Autodesk Fusion 360 part; units mm, degrees
note: some values were not read from the file. Chosen so that the rebuilt part matches the saved one: which face or edge a step refers to; which pieces of a blend or face edit are solid. Set by a fixed rule: which sketch regions a step uses.
(part 3 of 5)
sketch "スケッチ6" plane through (0, 0, 1.5) normal (0, 0, 1) x (-1, 0, 0)
  arc A0 (-32.0144, 97.3721) -> (-38.6662, 94.9272) centre (0, 0) ccw
  arc A1 (-26.3162, 95.431) -> (-32.0144, 97.3721) centre (-30.4528, 92.6222) ccw
  arc A2 (-26.3162, 95.431) -> (-25.9652, 94.9247) centre (0, 113.3) ccw
  arc A3 (-26.1835, 92.3551) -> (-25.9652, 94.9247) centre (-27.5978, 93.7693) ccw
  line L0 (-26.1835, 92.3551) -> (-32.3993, 86.1394)
  arc A4 (-35.2277, 86.1394) -> (-32.3993, 86.1394) centre (-33.8135, 87.5536) ccw
  line L1 (-35.2277, 86.1394) -> (-39.5548, 90.4665)
  arc A5 (-40.036, 92.519) -> (-39.5548, 90.4665) centre (-38.1406, 91.8807) ccw
  arc A6 (-40.036, 92.519) -> (-39.9088, 93.1825) centre (-42.4052, 93.3169) ccw
  arc A7 (-38.6662, 94.9272) -> (-39.9088, 93.1825) centre (-37.9117, 93.075) ccw
  line L2 (39.5548, 90.4665) -> (35.2277, 86.1394)
  arc A8 (32.3993, 86.1394) -> (35.2277, 86.1394) centre (33.8135, 87.5536) ccw
  line L3 (32.3993, 86.1394) -> (26.1835, 92.3551)
  arc A9 (25.9652, 94.9247) -> (26.1835, 92.3551) centre (27.5978, 93.7693) ccw
  arc A10 (25.9652, 94.9247) -> (26.3162, 95.431) centre (0, 113.3) ccw
  arc A11 (32.0144, 97.3721) -> (26.3162, 95.431) centre (30.4528, 92.6222) ccw
  arc A12 (38.6662, 94.9272) -> (32.0144, 97.3721) centre (0, 0) ccw
  arc A13 (39.9088, 93.1825) -> (38.6662, 94.9272) centre (37.9117, 93.075) ccw
  arc A14 (39.9088, 93.1825) -> (40.036, 92.519) centre (42.4052, 93.3169) ccw
  arc A15 (39.5548, 90.4665) -> (40.036, 92.519) centre (38.1406, 91.8807) ccw
  circle A16 centre (69.3456, -45.6575) radius 1.75
  circle A17 centre (-45.6575, -69.3456) radius 1.75
  circle A18 centre (-69.3456, 45.6575) radius 1.75
  circle A19 centre (69.3307, 45.6801) radius 1.75
  circle A20 centre (-93.3169, 42.4052) radius 1.75
  circle A21 centre (42.4052, -93.3169) radius 1.75
  circle A22 centre (93.3169, -42.4052) radius 1.75
  circle A23 centre (45.6801, -69.3307) radius 1.75
  circle A24 centre (-69.3307, -45.6801) radius 1.75
  circle A25 centre (-45.6801, 69.3307) radius 1.75
  circle A26 centre (45.6575, 69.3456) radius 1.75
  circle A27 centre (-93.3169, -42.4052) radius 1.75
  circle A28 centre (-42.4052, -93.3169) radius 1.75
  circle A29 centre (93.3169, 42.4052) radius 1.75
  circle A30 centre (39.2089, -15.5208) radius 1.75
  circle A31 centre (15.5208, -39.2089) radius 1.75
  circle A32 centre (26.1275, -49.8155) radius 1.75
  circle A33 centre (49.8155, -26.1275) radius 1.75
  circle A34 centre (-42.4052, 93.3169) radius 1.75
  circle A35 centre (-26.1275, 49.8155) radius 1.75
  arc A36 (-24.0851, 35.8083) -> (-23.3401, 43.4926) centre (-26.8756, 39.9571) ccw
  arc A37 (-24.0851, 35.8083) -> (-35.8083, 24.0851) centre (0, 0) ccw
  arc A38 (-43.4926, 23.3401) -> (-35.8083, 24.0851) centre (-39.9571, 26.8756) ccw
  line L4 (-43.4926, 23.3401) -> (-62.6322, 42.4797)
  arc A39 (-62.2927, 49.1749) -> (-62.6322, 42.4797) centre (-58.7571, 45.6394) ccw
  line L5 (-62.2927, 49.1749) -> (-49.1931, 62.2745)
  arc A40 (-42.122, 62.2745) -> (-49.1931, 62.2745) centre (-45.6575, 58.739) ccw
  line L6 (-42.122, 62.2745) -> (-23.3401, 43.4926)
  circle A41 centre (-49.8155, -26.1275) radius 1.75
  circle A42 centre (-49.8155, 26.1275) radius 1.75
  circle A43 centre (-15.5208, 39.2089) radius 1.75
  circle A44 centre (-26.1275, -49.8155) radius 1.75
  circle A45 centre (-39.2089, 15.5208) radius 1.75
  circle A46 centre (-15.5208, -39.2089) radius 1.75
  circle A47 centre (-39.2089, -15.5208) radius 1.75
  circle A48 centre (42.4052, 93.3169) radius 1.75
  arc A49 (17.125, 34.0956) -> (-17.125, 34.0956) centre (0, 0) ccw
  line L7 (17.125, 34.0956) -> (17.1965, 34.167)
  line L8 (17.1965, 34.167) -> (17.4152, 33.9483)
  arc A50 (33.9483, 17.4152) -> (17.4152, 33.9483) centre (0, 0) ccw
  line L9 (33.9483, 17.4152) -> (34.167, 17.1965)
  line L10 (34.167, 17.1965) -> (34.0956, 17.125)
  arc A51 (-34.0956, 17.125) -> (34.0956, 17.125) centre (0, 0) ccw
  line L11 (-34.0956, 17.125) -> (-34.167, 17.1965)
  line L12 (-34.167, 17.1965) -> (-33.9483, 17.4152)
  arc A52 (-17.4152, 33.9483) -> (-33.9483, 17.4152) centre (0, 0) ccw
  line L13 (-17.4152, 33.9483) -> (-17.1965, 34.167)
  line L14 (-17.1965, 34.167) -> (-17.125, 34.0956)
  line L15 (38.5865, 65.8101) -> (15.8059, 43.0296)
  arc A53 (10.9963, 41.7301) -> (15.8059, 43.0296) centre (12.2704, 46.5651) ccw
  arc A54 (10.9963, 41.7301) -> (-10.9963, 41.7301) centre (0, 0) ccw
  arc A55 (-15.8059, 43.0296) -> (-10.9963, 41.7301) centre (-12.2704, 46.5651) ccw
  line L16 (-15.8059, 43.0296) -> (-38.5865, 65.8101)
  arc A56 (-38.5865, 72.8811) -> (-38.5865, 65.8101) centre (-35.0509, 69.3456) ccw
  line L17 (-38.5865, 72.8811) -> (-24.7285, 86.7391)
  arc A57 (-18.3143, 87.2917) -> (-24.7285, 86.7391) centre (-21.193, 83.2035) ccw
  arc A58 (-18.3143, 87.2917) -> (18.3143, 87.2917) centre (0, 113.3) ccw
  arc A59 (24.7285, 86.7391) -> (18.3143, 87.2917) centre (21.193, 83.2035) ccw
  line L18 (24.7285, 86.7391) -> (38.5865, 72.8811)
  arc A60 (38.5865, 65.8101) -> (38.5865, 72.8811) centre (35.0509, 69.3456) ccw
  line L19 (62.6322, 42.4797) -> (43.4926, 23.3401)
  arc A61 (35.8083, 24.0851) -> (43.4926, 23.3401) centre (39.9571, 26.8756) ccw
  arc A62 (35.8083, 24.0851) -> (24.0851, 35.8083) centre (0, 0) ccw
  arc A63 (23.3401, 43.4926) -> (24.0851, 35.8083) centre (26.8756, 39.9571) ccw
  line L20 (23.3401, 43.4926) -> (42.122, 62.2745)
  arc A64 (49.1931, 62.2745) -> (42.122, 62.2745) centre (45.6575, 58.739) ccw
  line L21 (49.1931, 62.2745) -> (62.2927, 49.1749)
  arc A65 (62.6322, 42.4797) -> (62.2927, 49.1749) centre (58.7571, 45.6394) ccw
  arc A66 (91.4938, -47.061) -> (90.783, -46.7156) centre (91.0045, -47.1639) ccw
  arc A67 (91.4938, -47.061) -> (97.869, -44.4738) centre (93.3169, -42.4052) ccw
  arc A68 (97.869, -44.4738) -> (97.869, 44.4738) centre (0, 0) ccw
  arc A69 (97.869, 44.4738) -> (89.7814, 45.9408) centre (93.3169, 42.4052) ccw
  line L22 (89.7814, 45.9408) -> (84.7252, 40.8846)
  arc A70 (77.6541, 40.8846) -> (84.7252, 40.8846) centre (81.1896, 44.4201) ccw
  line L23 (77.6541, 40.8846) -> (40.8846, 77.6541)
  arc A71 (40.8846, 84.7252) -> (40.8846, 77.6541) centre (44.4201, 81.1896) ccw
  line L24 (40.8846, 84.7252) -> (45.9408, 89.7814)
  arc A72 (45.9408, 89.7814) -> (44.4738, 97.869) centre (42.4052, 93.3169) ccw
  arc A73 (44.4738, 97.869) -> (37.9262, 100.5876) centre (0, 0) ccw
  arc A74 (37.9256, 100.5859) -> (37.9262, 100.5876) centre (0, 113.3) ccw
  arc A75 (37.9256, 100.5859) -> (37.8014, 100.6345) centre (36.0432, 95.9538) ccw
  arc A76 (37.8014, 100.6345) -> (29.5575, 103.3567) centre (0, 0) ccw
  arc A77 (29.5575, 103.3567) -> (23.7528, 100.868) centre (28.1827, 98.5494) ccw
  arc A78 (-23.7528, 100.868) -> (23.7528, 100.868) centre (0, 113.3) ccw
  arc A79 (-23.7528, 100.868) -> (-29.5575, 103.3567) centre (-28.1827, 98.5494) ccw
  arc A80 (-29.5575, 103.3567) -> (-37.8014, 100.6345) centre (0, 0) ccw
  arc A81 (-37.8014, 100.6345) -> (-37.9256, 100.5859) centre (-36.0432, 95.9538) ccw
  arc A82 (-37.9262, 100.5876) -> (-37.9256, 100.5859) centre (0, 113.3) ccw
  arc A83 (-37.9262, 100.5876) -> (-44.4738, 97.869) centre (0, 0) ccw
  arc A84 (-44.4738, 97.869) -> (-45.9408, 89.7814) centre (-42.4052, 93.3169) ccw
  line L25 (-45.9408, 89.7814) -> (-40.8846, 84.7252)
  arc A85 (-40.8846, 77.6541) -> (-40.8846, 84.7252) centre (-44.4201, 81.1896) ccw
  line L26 (-40.8846, 77.6541) -> (-77.6541, 40.8846)
  arc A86 (-84.7252, 40.8846) -> (-77.6541, 40.8846) centre (-81.1896, 44.4201) ccw
  line L27 (-84.7252, 40.8846) -> (-89.7814, 45.9408)
  arc A87 (-89.7814, 45.9408) -> (-97.869, 44.4738) centre (-93.3169, 42.4052) ccw
  arc A88 (-97.869, 44.4738) -> (-97.869, -44.4738) centre (0, 0) ccw
  arc A89 (-97.869, -44.4738) -> (-91.4938, -47.061) centre (-93.3169, -42.4052) ccw
  arc A90 (-90.783, -46.7156) -> (-91.4938, -47.061) centre (-91.0045, -47.1639) ccw
  arc A91 (-90.783, -46.7156) -> (-89.7814, -45.9408) centre (-93.3169, -42.4052) ccw
  line L28 (-89.7814, -45.9408) -> (-84.7252, -40.8846)
  arc A92 (-77.6541, -40.8846) -> (-84.7252, -40.8846) centre (-81.1896, -44.4201) ccw
  line L29 (-77.6541, -40.8846) -> (-40.8846, -77.6541)
  arc A93 (-40.8846, -84.7252) -> (-40.8846, -77.6541) centre (-44.4201, -81.1896) ccw
  line L30 (-40.8846, -84.7252) -> (-45.9408, -89.7814)
  arc A94 (-45.9408, -89.7814) -> (-44.4738, -97.869) centre (-42.4052, -93.3169) ccw
  arc A95 (-44.4738, -97.869) -> (44.4738, -97.869) centre (0, 0) ccw
  arc A96 (44.4738, -97.869) -> (45.9408, -89.7814) centre (42.4052, -93.3169) ccw
  line L31 (45.9408, -89.7814) -> (40.8846, -84.7252)
  arc A97 (40.8846, -77.6541) -> (40.8846, -84.7252) centre (44.4201, -81.1896) ccw
  line L32 (40.8846, -77.6541) -> (77.6541, -40.8846)
  arc A98 (84.7252, -40.8846) -> (77.6541, -40.8846) centre (81.1896, -44.4201) ccw
  line L33 (84.7252, -40.8846) -> (89.7814, -45.9408)
  arc A99 (89.7814, -45.9408) -> (90.783, -46.7156) centre (93.3169, -42.4052) ccw
  circle A100 centre (49.8155, 26.1275) radius 1.75
  circle A101 centre (15.5208, 39.2089) radius 1.75
  circle A102 centre (39.2089, 15.5208) radius 1.75
  circle A103 centre (26.1275, 49.8155) radius 1.75
  line L34 (65.8101, -38.5865) -> (63.9577, -36.7341)
  line L35 (63.9577, -36.7341) -> (43.0296, -15.8059)
  arc A104 (41.7301, -10.9963) -> (43.0296, -15.8059) centre (46.5651, -12.2704) ccw
  arc A105 (41.7301, -10.9963) -> (41.7301, 10.9963) centre (0, 0) ccw
  arc A106 (43.0296, 15.8059) -> (41.7301, 10.9963) centre (46.5651, 12.2704) ccw
  line L36 (43.0296, 15.8059) -> (66.1678, 38.9441)
  arc A107 (72.863, 38.6046) -> (66.1678, 38.9441) centre (69.3275, 35.0691) ccw
  line L37 (72.863, 38.6046) -> (77.6541, 33.8135)
  arc A108 (77.6541, 33.8135) -> (84.7252, 33.8135) centre (81.1896, 37.349) ccw
  line L38 (84.7252, 33.8135) -> (88.0068, 37.0951)
  arc A109 (96.2368, 35.2806) -> (88.0068, 37.0951) centre (91.5424, 33.5596) ccw
  arc A110 (96.2368, -35.2806) -> (96.2368, 35.2806) centre (0, 0) ccw
  arc A111 (88.0068, -37.0951) -> (96.2368, -35.2806) centre (91.5424, -33.5596) ccw
  line L39 (88.0068, -37.0951) -> (84.7252, -33.8135)
  arc A112 (84.7252, -33.8135) -> (77.6541, -33.8135) centre (81.1896, -37.349) ccw
  line L40 (77.6541, -33.8135) -> (72.8811, -38.5865)
  arc A113 (65.8101, -38.5865) -> (72.8811, -38.5865) centre (69.3456, -35.0509) ccw
  arc A114 (42.4797, -62.6322) -> (49.1749, -62.2927) centre (45.6394, -58.7571) ccw
  line L41 (42.4797, -62.6322) -> (23.3401, -43.4926)
  arc A115 (24.0851, -35.8083) -> (23.3401, -43.4926) centre (26.8756, -39.9571) ccw
  arc A116 (24.0851, -35.8083) -> (35.8083, -24.0851) centre (0, 0) ccw
  arc A117 (43.4926, -23.3401) -> (35.8083, -24.0851) centre (39.9571, -26.8756) ccw
  line L42 (43.4926, -23.3401) -> (62.2745, -42.122)
  arc A118 (62.2745, -49.1931) -> (62.2745, -42.122) centre (58.739, -45.6575) ccw
  line L43 (62.2745, -49.1931) -> (49.1749, -62.2927)
  arc A119 (-77.6541, -33.8135) -> (-84.7252, -33.8135) centre (-81.1896, -37.349) ccw
  line L44 (-84.7252, -33.8135) -> (-88.0068, -37.0951)
  arc A120 (-96.2368, -35.2806) -> (-88.0068, -37.0951) centre (-91.5424, -33.5596) ccw
  arc A121 (-96.2368, 35.2806) -> (-96.2368, -35.2806) centre (0, 0) ccw
  arc A122 (-88.0068, 37.0951) -> (-96.2368, 35.2806) centre (-91.5424, 33.5596) ccw
  line L45 (-88.0068, 37.0951) -> (-84.7252, 33.8135)
  arc A123 (-84.7252, 33.8135) -> (-77.6541, 33.8135) centre (-81.1896, 37.349) ccw
  line L46 (-77.6541, 33.8135) -> (-72.863, 38.6046)
  arc A124 (-66.1678, 38.9441) -> (-72.863, 38.6046) centre (-69.3275, 35.0691) ccw
  line L47 (-66.1678, 38.9441) -> (-43.0296, 15.8059)
  arc A125 (-41.7301, 10.9963) -> (-43.0296, 15.8059) centre (-46.5651, 12.2704) ccw
  arc A126 (-41.7301, 10.9963) -> (-41.7301, -10.9963) centre (0, 0) ccw
  arc A127 (-43.0296, -15.8059) -> (-41.7301, -10.9963) centre (-46.5651, -12.2704) ccw
  line L48 (-43.0296, -15.8059) -> (-63.9577, -36.7341)
  line L49 (-63.9577, -36.7341) -> (-66.1678, -38.9441)
  arc A128 (-72.863, -38.6046) -> (-66.1678, -38.9441) centre (-69.3275, -35.0691) ccw
  line L50 (-72.863, -38.6046) -> (-77.6541, -33.8135)
  arc A129 (29.6417, -59.2224) -> (32.277, -61.8576) centre (32.1379, -59.3615) ccw
  arc A130 (36.0907, -63.3143) -> (32.277, -61.8576) centre (32.5552, -66.8499) ccw
  line L51 (36.0907, -63.3143) -> (38.9441, -66.1678)
  arc A131 (38.6046, -72.863) -> (38.9441, -66.1678) centre (35.0691, -69.3275) ccw
  line L52 (38.6046, -72.863) -> (33.8146, -77.653)
  arc A132 (33.8146, -77.653) -> (33.7038, -84.612) centre (37.349, -81.1896) ccw
  line L53 (33.7038, -84.612) -> (33.8135, -84.7252)
  line L54 (33.8135, -84.7252) -> (37.0951, -88.0068)
  arc A133 (35.2806, -96.2368) -> (37.0951, -88.0068) centre (33.5596, -91.5424) ccw
  arc A134 (-35.2806, -96.2368) -> (35.2806, -96.2368) centre (0, 0) ccw
  arc A135 (-37.0951, -88.0068) -> (-35.2806, -96.2368) centre (-33.5596, -91.5424) ccw
  line L55 (-37.0951, -88.0068) -> (-33.8135, -84.7252)
  line L56 (-33.8135, -84.7252) -> (-33.7586, -84.6686)
  arc A136 (-33.7586, -84.6686) -> (-33.8139, -77.6537) centre (-37.3495, -81.1892) ccw
  line L57 (-33.8139, -77.6537) -> (-38.5865, -72.8811)
  arc A137 (-38.9491, -66.2144) -> (-38.5865, -72.8811) centre (-35.0509, -69.3456) ccw
  arc A138 (-38.9441, -66.1678) -> (-38.9491, -66.2144) centre (-33.9744, -66.7173) ccw
  line L58 (-38.9441, -66.1678) -> (-36.0907, -63.3143)
  arc A139 (-32.277, -61.8576) -> (-36.0907, -63.3143) centre (-32.5552, -66.8499) ccw
  arc A140 (-32.277, -61.8576) -> (-29.6417, -59.2224) centre (-32.1379, -59.3615) ccw
  arc A141 (-28.185, -55.4086) -> (-29.6417, -59.2224) centre (-24.6495, -58.9442) ccw
  line L59 (-28.185, -55.4086) -> (-15.8059, -43.0296)
  arc A142 (-10.9963, -41.7301) -> (-15.8059, -43.0296) centre (-12.2704, -46.5651) ccw
  arc A143 (-10.9963, -41.7301) -> (10.9963, -41.7301) centre (0, 0) ccw
  arc A144 (15.8059, -43.0296) -> (10.9963, -41.7301) centre (12.2704, -46.5651) ccw
  line L60 (15.8059, -43.0296) -> (28.185, -55.4086)
  arc A145 (29.6417, -59.2224) -> (28.185, -55.4086) centre (24.6495, -58.9442) ccw
  arc A146 (-62.6322, -42.4797) -> (-62.2927, -49.1749) centre (-58.7571, -45.6394) ccw
  line L61 (-62.6322, -42.4797) -> (-43.4926, -23.3401)
  arc A147 (-35.8083, -24.0851) -> (-43.4926, -23.3401) centre (-39.9571, -26.8756) ccw
  arc A148 (-35.8083, -24.0851) -> (-24.0851, -35.8083) centre (0, 0) ccw
  arc A149 (-23.3401, -43.4926) -> (-24.0851, -35.8083) centre (-26.8756, -39.9571) ccw
  line L62 (-23.3401, -43.4926) -> (-42.122, -62.2745)
  arc A150 (-49.1931, -62.2745) -> (-42.122, -62.2745) centre (-45.6575, -58.739) ccw
  line L63 (-49.1931, -62.2745) -> (-62.2927, -49.1749)
  circle A151 centre (-32.1379, -59.3615) radius 1.75
  circle A152 centre (32.1379, -59.3615) radius 1.75
  circle A153 centre (93.3169, -42.4052) radius 1.75
  arc A154 (52.3726, -91.0061) -> (91.0061, -52.3726) centre (0, 0) ccw
  arc A155 (93.6969, 47.3908) -> (-47.3908, -93.6969) centre (0, 0) ccw
  arc A156 (44.4738, -97.869) -> (97.869, -44.4738) centre (0, 0) ccw
  arc A157 (97.869, 44.4738) -> (-44.4738, -97.869) centre (0, 0) ccw
  arc A158 (46.1419, -89.9947) -> (44.4738, -97.869) centre (42.4052, -93.3169) ccw
  arc A159 (97.869, -44.4738) -> (89.9947, -46.1419) centre (93.3169, -42.4052) ccw
  arc A160 (46.1419, -89.9947) -> (52.3726, -91.0061) centre (49.8786, -86.6725) ccw
  arc A161 (91.0061, -52.3726) -> (89.9947, -46.1419) centre (86.6725, -49.8786) ccw
  arc A162 (91.0061, -52.3726) -> (89.9947, -46.1419) centre (86.6725, -49.8786) ccw
  arc A163 (46.1419, -89.9947) -> (52.3726, -91.0061) centre (49.8786, -86.6725) ccw
  circle A164 centre (93.3169, -42.4052) radius 1.75
  arc A165 (46.1419, -89.9947) -> (44.4738, -97.869) centre (42.4052, -93.3169) ccw
  arc A166 (97.869, -44.4738) -> (89.9947, -46.1419) centre (93.3169, -42.4052) ccw
  arc A167 (44.4738, -97.869) -> (97.869, -44.4738) centre (0, 0) ccw
  arc A168 (52.3726, -91.0061) -> (91.0061, -52.3726) centre (0, 0) ccw
  circle A169 centre (33.5596, -91.5424) radius 5
  circle A170 centre (91.5424, -33.5596) radius 5
  circle A171 centre (42.4052, -93.3169) radius 1.75
  circle A172 centre (91.5424, -33.5596) radius 5
  circle A173 centre (33.5596, -91.5424) radius 5
  arc A174 (44.4738, -97.869) -> (97.869, -44.4738) centre (0, 0) ccw
  arc A175 (46.1419, -89.9947) -> (44.4738, -97.869) centre (42.4052, -93.3169) ccw
  arc A176 (97.869, -44.4738) -> (89.9947, -46.1419) centre (93.3169, -42.4052) ccw
  circle A177 centre (93.3169, -42.4052) radius 1.75
  arc A178 (44.4738, -97.869) -> (97.869, -44.4738) centre (0, 0) ccw
  arc A179 (97.869, -44.4738) -> (89.9947, -46.1419) centre (93.3169, -42.4052) ccw
  arc A180 (52.3726, -91.0061) -> (91.0061, -52.3726) centre (0, 0) ccw
  arc A181 (46.1419, -89.9947) -> (44.4738, -97.869) centre (42.4052, -93.3169) ccw
  arc A182 (91.0061, -52.3726) -> (89.9947, -46.1419) centre (86.6725, -49.8786) ccw
  circle A183 centre (93.3169, -42.4052) radius 1.75
  arc A184 (46.1419, -89.9947) -> (52.3726, -91.0061) centre (49.8786, -86.6725) ccw
  arc A185 (91.0061, -52.3726) -> (89.9947, -46.1419) centre (86.6725, -49.8786) ccw
  circle A186 centre (42.4052, -93.3169) radius 1.75
  arc A187 (46.1419, -89.9947) -> (52.3726, -91.0061) centre (49.8786, -86.6725) ccw
  arc A188 (52.3726, -91.0061) -> (91.0061, -52.3726) centre (0, 0) ccw
  point P0 (93.6969, 47.3908)
  dimension "d116" = 5
  dimension "d117" = 5
  dimension "d118" = 5
  dimension "d119" = 5
  dimension "d120" = 5
  dimension "d121" = 5
  dimension "d122" = 5
  dimension "d123" = 5
  constraint concentric A0 A156
  constraint concentric A0 A154
  constraint concentric A22 A153
  constraint concentric A22 A159
  constraint concentric A21 A158
  constraint coincident A94 A155.end
  constraint coincident A69 P0
  constraint concentric A154 A155
  constraint concentric A156 A157
  constraint tangent A158 A160
  constraint tangent A154 A160
  constraint tangent A159 A161
  constraint tangent A154 A161
  constraint tangent A163 A165
  constraint tangent A163 A168
  constraint tangent A162 A166
  constraint tangent A162 A168
  constraint concentric A133 A169
  constraint concentric A111 A170
  constraint concentric A158 A171
  constraint tangent A175 A187
  constraint tangent A180 A187
  constraint tangent A176 A182
  constraint tangent A180 A182
  constraint tangent A181 A184
  constraint tangent A184 A188
  constraint tangent A179 A185
  constraint tangent A185 A188
  constraint concentric A175 A186
  measures "d116" radius of A160
  measures "d117" radius of A161
  measures "d118" radius of A163
  measures "d119" radius of A162
  measures "d120" radius of A187
  measures "d121" radius of A182
  measures "d122" radius of A184
  measures "d123" radius of A185
sketch "スケッチ7" plane through (0, 0, 1.5) normal (0, 0, 1) x (-1, 0, 0)
  arc A0 (-32.0144, 97.3721) -> (-38.6662, 94.9272) centre (0, 0) ccw
  arc A1 (-26.3162, 95.431) -> (-32.0144, 97.3721) centre (-30.4528, 92.6222) ccw
  arc A2 (-26.3162, 95.431) -> (-25.9652, 94.9247) centre (0, 113.3) ccw
  arc A3 (-26.1835, 92.3551) -> (-25.9652, 94.9247) centre (-27.5978, 93.7693) ccw
  line L0 (-26.1835, 92.3551) -> (-32.3993, 86.1394)
  arc A4 (-35.2277, 86.1394) -> (-32.3993, 86.1394) centre (-33.8135, 87.5536) ccw
  line L1 (-35.2277, 86.1394) -> (-39.5548, 90.4665)
  arc A5 (-40.036, 92.519) -> (-39.5548, 90.4665) centre (-38.1406, 91.8807) ccw
  arc A6 (-40.036, 92.519) -> (-39.9088, 93.1825) centre (-42.4052, 93.3169) ccw
  arc A7 (-38.6662, 94.9272) -> (-39.9088, 93.1825) centre (-37.9117, 93.075) ccw
  line L2 (39.5548, 90.4665) -> (35.2277, 86.1394)
  arc A8 (32.3993, 86.1394) -> (35.2277, 86.1394) centre (33.8135, 87.5536) ccw
  line L3 (32.3993, 86.1394) -> (26.1835, 92.3551)
  arc A9 (25.9652, 94.9247) -> (26.1835, 92.3551) centre (27.5978, 93.7693) ccw
  arc A10 (25.9652, 94.9247) -> (26.3162, 95.431) centre (0, 113.3) ccw
  arc A11 (32.0144, 97.3721) -> (26.3162, 95.431) centre (30.4528, 92.6222) ccw
  arc A12 (38.6662, 94.9272) -> (32.0144, 97.3721) centre (0, 0) ccw
  arc A13 (39.9088, 93.1825) -> (38.6662, 94.9272) centre (37.9117, 93.075) ccw
  arc A14 (39.9088, 93.1825) -> (40.036, 92.519) centre (42.4052, 93.3169) ccw
  arc A15 (39.5548, 90.4665) -> (40.036, 92.519) centre (38.1406, 91.8807) ccw
  circle A16 centre (69.3456, -45.6575) radius 1.75
  circle A17 centre (-45.6575, -69.3456) radius 1.75
  circle A18 centre (-69.3456, 45.6575) radius 1.75
  circle A19 centre (69.3307, 45.6801) radius 1.75
  circle A20 centre (-93.3169, 42.4052) radius 1.75
  circle A21 centre (42.4052, -93.3169) radius 1.75
  circle A22 centre (93.3169, -42.4052) radius 1.75
  circle A23 centre (45.6801, -69.3307) radius 1.75
  circle A24 centre (-69.3307, -45.6801) radius 1.75
  circle A25 centre (-45.6801, 69.3307) radius 1.75
  circle A26 centre (45.6575, 69.3456) radius 1.75
  circle A27 centre (-93.3169, -42.4052) radius 1.75
  circle A28 centre (-42.4052, -93.3169) radius 1.75
  circle A29 centre (93.3169, 42.4052) radius 1.75
  circle A30 centre (39.2089, -15.5208) radius 1.75
  circle A31 centre (15.5208, -39.2089) radius 1.75
  circle A32 centre (26.1275, -49.8155) radius 1.75
  circle A33 centre (49.8155, -26.1275) radius 1.75
  circle A34 centre (-42.4052, 93.3169) radius 1.75
  circle A35 centre (-26.1275, 49.8155) radius 1.75
  arc A36 (-24.0851, 35.8083) -> (-23.3401, 43.4926) centre (-26.8756, 39.9571) ccw
  arc A37 (-24.0851, 35.8083) -> (-35.8083, 24.0851) centre (0, 0) ccw
  arc A38 (-43.4926, 23.3401) -> (-35.8083, 24.0851) centre (-39.9571, 26.8756) ccw
  line L4 (-43.4926, 23.3401) -> (-62.6322, 42.4797)
  arc A39 (-62.2927, 49.1749) -> (-62.6322, 42.4797) centre (-58.7571, 45.6394) ccw
  line L5 (-62.2927, 49.1749) -> (-49.1931, 62.2745)
  arc A40 (-42.122, 62.2745) -> (-49.1931, 62.2745) centre (-45.6575, 58.739) ccw
  line L6 (-42.122, 62.2745) -> (-23.3401, 43.4926)
  circle A41 centre (-49.8155, -26.1275) radius 1.75
  circle A42 centre (-49.8155, 26.1275) radius 1.75
  circle A43 centre (-15.5208, 39.2089) radius 1.75
  circle A44 centre (-26.1275, -49.8155) radius 1.75
  circle A45 centre (-39.2089, 15.5208) radius 1.75
  circle A46 centre (-15.5208, -39.2089) radius 1.75
  circle A47 centre (-39.2089, -15.5208) radius 1.75
  circle A48 centre (42.4052, 93.3169) radius 1.75
  arc A49 (17.125, 34.0956) -> (-17.125, 34.0956) centre (0, 0) ccw
  line L7 (17.125, 34.0956) -> (17.1965, 34.167)
  line L8 (17.1965, 34.167) -> (17.4152, 33.9483)
  arc A50 (33.9483, 17.4152) -> (17.4152, 33.9483) centre (0, 0) ccw
  line L9 (33.9483, 17.4152) -> (34.167, 17.1965)
  line L10 (34.167, 17.1965) -> (34.0956, 17.125)
  arc A51 (-34.0956, 17.125) -> (34.0956, 17.125) centre (0, 0) ccw
  line L11 (-34.0956, 17.125) -> (-34.167, 17.1965)
  line L12 (-34.167, 17.1965) -> (-33.9483, 17.4152)
  arc A52 (-17.4152, 33.9483) -> (-33.9483, 17.4152) centre (0, 0) ccw
  line L13 (-17.4152, 33.9483) -> (-17.1965, 34.167)
  line L14 (-17.1965, 34.167) -> (-17.125, 34.0956)
  line L15 (38.5865, 65.8101) -> (15.8059, 43.0296)
  arc A53 (10.9963, 41.7301) -> (15.8059, 43.0296) centre (12.2704, 46.5651) ccw
  arc A54 (10.9963, 41.7301) -> (-10.9963, 41.7301) centre (0, 0) ccw
  arc A55 (-15.8059, 43.0296) -> (-10.9963, 41.7301) centre (-12.2704, 46.5651) ccw
  line L16 (-15.8059, 43.0296) -> (-38.5865, 65.8101)
  arc A56 (-38.5865, 72.8811) -> (-38.5865, 65.8101) centre (-35.0509, 69.3456) ccw
  line L17 (-38.5865, 72.8811) -> (-24.7285, 86.7391)
  arc A57 (-18.3143, 87.2917) -> (-24.7285, 86.7391) centre (-21.193, 83.2035) ccw
  arc A58 (-18.3143, 87.2917) -> (18.3143, 87.2917) centre (0, 113.3) ccw
  arc A59 (24.7285, 86.7391) -> (18.3143, 87.2917) centre (21.193, 83.2035) ccw
  line L18 (24.7285, 86.7391) -> (38.5865, 72.8811)
  arc A60 (38.5865, 65.8101) -> (38.5865, 72.8811) centre (35.0509, 69.3456) ccw
  line L19 (62.6322, 42.4797) -> (43.4926, 23.3401)
  arc A61 (35.8083, 24.0851) -> (43.4926, 23.3401) centre (39.9571, 26.8756) ccw
  arc A62 (35.8083, 24.0851) -> (24.0851, 35.8083) centre (0, 0) ccw
  arc A63 (23.3401, 43.4926) -> (24.0851, 35.8083) centre (26.8756, 39.9571) ccw
  line L20 (23.3401, 43.4926) -> (42.122, 62.2745)
  arc A64 (49.1931, 62.2745) -> (42.122, 62.2745) centre (45.6575, 58.739) ccw
  line L21 (49.1931, 62.2745) -> (62.2927, 49.1749)
  arc A65 (62.6322, 42.4797) -> (62.2927, 49.1749) centre (58.7571, 45.6394) ccw
  arc A66 (91.4938, -47.061) -> (90.783, -46.7156) centre (91.0045, -47.1639) ccw
  arc A67 (91.4938, -47.061) -> (97.869, -44.4738) centre (93.3169, -42.4052) ccw
  arc A68 (97.869, -44.4738) -> (97.869, 44.4738) centre (0, 0) ccw
  arc A69 (97.869, 44.4738) -> (89.7814, 45.9408) centre (93.3169, 42.4052) ccw
  line L22 (89.7814, 45.9408) -> (84.7252, 40.8846)
  arc A70 (77.6541, 40.8846) -> (84.7252, 40.8846) centre (81.1896, 44.4201) ccw
  line L23 (77.6541, 40.8846) -> (40.8846, 77.6541)
  arc A71 (40.8846, 84.7252) -> (40.8846, 77.6541) centre (44.4201, 81.1896) ccw
  line L24 (40.8846, 84.7252) -> (45.9408, 89.7814)
  arc A72 (45.9408, 89.7814) -> (44.4738, 97.869) centre (42.4052, 93.3169) ccw
  arc A73 (44.4738, 97.869) -> (37.9262, 100.5876) centre (0, 0) ccw
  arc A74 (37.9256, 100.5859) -> (37.9262, 100.5876) centre (0, 113.3) ccw
  arc A75 (37.9256, 100.5859) -> (37.8014, 100.6345) centre (36.0432, 95.9538) ccw
  arc A76 (37.8014, 100.6345) -> (29.5575, 103.3567) centre (0, 0) ccw
  arc A77 (29.5575, 103.3567) -> (23.7528, 100.868) centre (28.1827, 98.5494) ccw
  arc A78 (-23.7528, 100.868) -> (23.7528, 100.868) centre (0, 113.3) ccw
  arc A79 (-23.7528, 100.868) -> (-29.5575, 103.3567) centre (-28.1827, 98.5494) ccw
  arc A80 (-29.5575, 103.3567) -> (-37.8014, 100.6345) centre (0, 0) ccw
  arc A81 (-37.8014, 100.6345) -> (-37.9256, 100.5859) centre (-36.0432, 95.9538) ccw
  arc A82 (-37.9262, 100.5876) -> (-37.9256, 100.5859) centre (0, 113.3) ccw
  arc A83 (-37.9262, 100.5876) -> (-44.4738, 97.869) centre (0, 0) ccw
  arc A84 (-44.4738, 97.869) -> (-45.9408, 89.7814) centre (-42.4052, 93.3169) ccw
  line L25 (-45.9408, 89.7814) -> (-40.8846, 84.7252)
  arc A85 (-40.8846, 77.6541) -> (-40.8846, 84.7252) centre (-44.4201, 81.1896) ccw
  line L26 (-40.8846, 77.6541) -> (-77.6541, 40.8846)
  arc A86 (-84.7252, 40.8846) -> (-77.6541, 40.8846) centre (-81.1896, 44.4201) ccw
  line L27 (-84.7252, 40.8846) -> (-89.7814, 45.9408)
  arc A87 (-89.7814, 45.9408) -> (-97.869, 44.4738) centre (-93.3169, 42.4052) ccw
  arc A88 (-97.869, 44.4738) -> (-97.869, -44.4738) centre (0, 0) ccw
  arc A89 (-97.869, -44.4738) -> (-91.4938, -47.061) centre (-93.3169, -42.4052) ccw
  arc A90 (-90.783, -46.7156) -> (-91.4938, -47.061) centre (-91.0045, -47.1639) ccw
  arc A91 (-90.783, -46.7156) -> (-89.7814, -45.9408) centre (-93.3169, -42.4052) ccw
  line L28 (-89.7814, -45.9408) -> (-84.7252, -40.8846)
  arc A92 (-77.6541, -40.8846) -> (-84.7252, -40.8846) centre (-81.1896, -44.4201) ccw
  line L29 (-77.6541, -40.8846) -> (-40.8846, -77.6541)
  arc A93 (-40.8846, -84.7252) -> (-40.8846, -77.6541) centre (-44.4201, -81.1896) ccw
  line L30 (-40.8846, -84.7252) -> (-45.9408, -89.7814)
  arc A94 (-45.9408, -89.7814) -> (-44.4738, -97.869) centre (-42.4052, -93.3169) ccw
  arc A95 (-44.4738, -97.869) -> (44.4738, -97.869) centre (0, 0) ccw
  arc A96 (44.4738, -97.869) -> (45.9408, -89.7814) centre (42.4052, -93.3169) ccw
  line L31 (45.9408, -89.7814) -> (40.8846, -84.7252)
  arc A97 (40.8846, -77.6541) -> (40.8846, -84.7252) centre (44.4201, -81.1896) ccw
  line L32 (40.8846, -77.6541) -> (77.6541, -40.8846)
  arc A98 (84.7252, -40.8846) -> (77.6541, -40.8846) centre (81.1896, -44.4201) ccw
  line L33 (84.7252, -40.8846) -> (89.7814, -45.9408)
  arc A99 (89.7814, -45.9408) -> (90.783, -46.7156) centre (93.3169, -42.4052) ccw
  circle A100 centre (49.8155, 26.1275) radius 1.75
  circle A101 centre (15.5208, 39.2089) radius 1.75
  circle A102 centre (39.2089, 15.5208) radius 1.75
  circle A103 centre (26.1275, 49.8155) radius 1.75
  line L34 (65.8101, -38.5865) -> (63.9577, -36.7341)
  line L35 (63.9577, -36.7341) -> (43.0296, -15.8059)
  arc A104 (41.7301, -10.9963) -> (43.0296, -15.8059) centre (46.5651, -12.2704) ccw
  arc A105 (41.7301, -10.9963) -> (41.7301, 10.9963) centre (0, 0) ccw
  arc A106 (43.0296, 15.8059) -> (41.7301, 10.9963) centre (46.5651, 12.2704) ccw
  line L36 (43.0296, 15.8059) -> (66.1678, 38.9441)
  arc A107 (72.863, 38.6046) -> (66.1678, 38.9441) centre (69.3275, 35.0691) ccw
  line L37 (72.863, 38.6046) -> (77.6541, 33.8135)
  arc A108 (77.6541, 33.8135) -> (84.7252, 33.8135) centre (81.1896, 37.349) ccw
  line L38 (84.7252, 33.8135) -> (88.0068, 37.0951)
  arc A109 (96.2368, 35.2806) -> (88.0068, 37.0951) centre (91.5424, 33.5596) ccw
  arc A110 (96.2368, -35.2806) -> (96.2368, 35.2806) centre (0, 0) ccw
  arc A111 (88.0068, -37.0951) -> (96.2368, -35.2806) centre (91.5424, -33.5596) ccw
  line L39 (88.0068, -37.0951) -> (84.7252, -33.8135)
  arc A112 (84.7252, -33.8135) -> (77.6541, -33.8135) centre (81.1896, -37.349) ccw
  line L40 (77.6541, -33.8135) -> (72.8811, -38.5865)
  arc A113 (65.8101, -38.5865) -> (72.8811, -38.5865) centre (69.3456, -35.0509) ccw
  arc A114 (42.4797, -62.6322) -> (49.1749, -62.2927) centre (45.6394, -58.7571) ccw
  line L41 (42.4797, -62.6322) -> (23.3401, -43.4926)
  arc A115 (24.0851, -35.8083) -> (23.3401, -43.4926) centre (26.8756, -39.9571) ccw
  arc A116 (24.0851, -35.8083) -> (35.8083, -24.0851) centre (0, 0) ccw
  arc A117 (43.4926, -23.3401) -> (35.8083, -24.0851) centre (39.9571, -26.8756) ccw
  line L42 (43.4926, -23.3401) -> (62.2745, -42.122)
  arc A118 (62.2745, -49.1931) -> (62.2745, -42.122) centre (58.739, -45.6575) ccw
  line L43 (62.2745, -49.1931) -> (49.1749, -62.2927)
  arc A119 (-77.6541, -33.8135) -> (-84.7252, -33.8135) centre (-81.1896, -37.349) ccw
  line L44 (-84.7252, -33.8135) -> (-88.0068, -37.0951)
  arc A120 (-96.2368, -35.2806) -> (-88.0068, -37.0951) centre (-91.5424, -33.5596) ccw
  arc A121 (-96.2368, 35.2806) -> (-96.2368, -35.2806) centre (0, 0) ccw
  arc A122 (-88.0068, 37.0951) -> (-96.2368, 35.2806) centre (-91.5424, 33.5596) ccw
  line L45 (-88.0068, 37.0951) -> (-84.7252, 33.8135)
  arc A123 (-84.7252, 33.8135) -> (-77.6541, 33.8135) centre (-81.1896, 37.349) ccw
  line L46 (-77.6541, 33.8135) -> (-72.863, 38.6046)
  arc A124 (-66.1678, 38.9441) -> (-72.863, 38.6046) centre (-69.3275, 35.0691) ccw
  line L47 (-66.1678, 38.9441) -> (-43.0296, 15.8059)
  arc A125 (-41.7301, 10.9963) -> (-43.0296, 15.8059) centre (-46.5651, 12.2704) ccw
  arc A126 (-41.7301, 10.9963) -> (-41.7301, -10.9963) centre (0, 0) ccw
  arc A127 (-43.0296, -15.8059) -> (-41.7301, -10.9963) centre (-46.5651, -12.2704) ccw
  line L48 (-43.0296, -15.8059) -> (-63.9577, -36.7341)
  line L49 (-63.9577, -36.7341) -> (-66.1678, -38.9441)
  arc A128 (-72.863, -38.6046) -> (-66.1678, -38.9441) centre (-69.3275, -35.0691) ccw
  line L50 (-72.863, -38.6046) -> (-77.6541, -33.8135)
  arc A129 (29.6417, -59.2224) -> (32.277, -61.8576) centre (32.1379, -59.3615) ccw
  arc A130 (36.0907, -63.3143) -> (32.277, -61.8576) centre (32.5552, -66.8499) ccw
  line L51 (36.0907, -63.3143) -> (38.9441, -66.1678)
  arc A131 (38.6046, -72.863) -> (38.9441, -66.1678) centre (35.0691, -69.3275) ccw
  line L52 (38.6046, -72.863) -> (33.8146, -77.653)
  arc A132 (33.8146, -77.653) -> (33.7038, -84.612) centre (37.349, -81.1896) ccw
  line L53 (33.7038, -84.612) -> (33.8135, -84.7252)
  line L54 (33.8135, -84.7252) -> (37.0951, -88.0068)
  arc A133 (35.2806, -96.2368) -> (37.0951, -88.0068) centre (33.5596, -91.5424) ccw
  arc A134 (-35.2806, -96.2368) -> (35.2806, -96.2368) centre (0, 0) ccw
  arc A135 (-37.0951, -88.0068) -> (-35.2806, -96.2368) centre (-33.5596, -91.5424) ccw
  line L55 (-37.0951, -88.0068) -> (-33.8135, -84.7252)
  line L56 (-33.8135, -84.7252) -> (-33.7586, -84.6686)
  arc A136 (-33.7586, -84.6686) -> (-33.8139, -77.6537) centre (-37.3495, -81.1892) ccw
  line L57 (-33.8139, -77.6537) -> (-38.5865, -72.8811)
  arc A137 (-38.9491, -66.2144) -> (-38.5865, -72.8811) centre (-35.0509, -69.3456) ccw
  arc A138 (-38.9441, -66.1678) -> (-38.9491, -66.2144) centre (-33.9744, -66.7173) ccw
  line L58 (-38.9441, -66.1678) -> (-36.0907, -63.3143)
  arc A139 (-32.277, -61.8576) -> (-36.0907, -63.3143) centre (-32.5552, -66.8499) ccw
  arc A140 (-32.277, -61.8576) -> (-29.6417, -59.2224) centre (-32.1379, -59.3615) ccw
  arc A141 (-28.185, -55.4086) -> (-29.6417, -59.2224) centre (-24.6495, -58.9442) ccw
  line L59 (-28.185, -55.4086) -> (-15.8059, -43.0296)
  arc A142 (-10.9963, -41.7301) -> (-15.8059, -43.0296) centre (-12.2704, -46.5651) ccw
  arc A143 (-10.9963, -41.7301) -> (10.9963, -41.7301) centre (0, 0) ccw
  arc A144 (15.8059, -43.0296) -> (10.9963, -41.7301) centre (12.2704, -46.5651) ccw
  line L60 (15.8059, -43.0296) -> (28.185, -55.4086)
  arc A145 (29.6417, -59.2224) -> (28.185, -55.4086) centre (24.6495, -58.9442) ccw
  arc A146 (-62.6322, -42.4797) -> (-62.2927, -49.1749) centre (-58.7571, -45.6394) ccw
  line L61 (-62.6322, -42.4797) -> (-43.4926, -23.3401)
  arc A147 (-35.8083, -24.0851) -> (-43.4926, -23.3401) centre (-39.9571, -26.8756) ccw
  arc A148 (-35.8083, -24.0851) -> (-24.0851, -35.8083) centre (0, 0) ccw
  arc A149 (-23.3401, -43.4926) -> (-24.0851, -35.8083) centre (-26.8756, -39.9571) ccw
  line L62 (-23.3401, -43.4926) -> (-42.122, -62.2745)
  arc A150 (-49.1931, -62.2745) -> (-42.122, -62.2745) centre (-45.6575, -58.739) ccw
  line L63 (-49.1931, -62.2745) -> (-62.2927, -49.1749)
  circle A151 centre (-32.1379, -59.3615) radius 1.75
  circle A152 centre (32.1379, -59.3615) radius 1.75
  line L64 (80.8769, 30.5907) -> (81.1896, 30.278)
  arc A153 (77.6541, 33.8135) -> (84.7252, 33.8135) centre (81.1896, 37.349) ccw
  circle A154 centre (51.6679, 27.9799) radius 1.75
  line L65 (33.8135, 16.8429) -> (34.167, 17.1965)
  arc A155 (84.7252, -33.8135) -> (77.6541, -33.8135) centre (81.1896, -37.349) ccw
  line L66 (92.8569, -49.0163) -> (84.7252, -40.8846)
  line L67 (92.8569, -49.0163) -> (84.7252, -40.8846)
  arc A156 (88.0068, -37.0951) -> (96.2368, -35.2806) centre (91.5424, -33.5596) ccw
  arc A157 (89.7814, -45.9408) -> (97.869, -44.4738) centre (93.3169, -42.4052) ccw
  arc A158 (84.7252, -33.8135) -> (77.6541, -33.8135) centre (81.1896, -37.349) ccw
  line L68 (92.8569, -49.0163) -> (85.4323, -41.5917)
  arc A159 (89.7814, -45.9408) -> (97.869, -44.4738) centre (93.3169, -42.4052) ccw
  line L69 (68.8153, -49.7234) -> (77.6541, -40.8846)
  line L70 (92.8569, -49.0163) -> (86.6476, -42.807)
  line L71 (92.8569, -49.0163) -> (85.4323, -41.5917)
  arc A160 (84.7252, -40.8846) -> (77.6541, -40.8846) centre (81.1896, -44.4201) ccw
  line L72 (84.7252, -33.8135) -> (88.0068, -37.0951)
  line L73 (92.8569, -49.0163) -> (89.7814, -45.9408)
  line L74 (92.8569, -49.0163) -> (89.7814, -45.9408)
  line L75 (84.7252, -33.8135) -> (88.0068, -37.0951)
  arc A161 (84.7252, -40.8846) -> (77.6541, -40.8846) centre (81.1896, -44.4201) ccw
  line L76 (68.8153, -49.7234) -> (77.6541, -40.8846)
  arc A162 (86.6476, -42.807) -> (99.7259, -40.1371) centre (92.3045, -37.1501) ccw
  arc A163 (88.0068, -37.0951) -> (96.2368, -35.2806) centre (91.5424, -33.5596) ccw
  circle A164 centre (41.0613, -17.3733) radius 1.75
  line L77 (29.2173, -57.5016) -> (11.5396, -39.8239)
  line L78 (34.167, -17.1965) -> (33.8135, -16.8429)
  circle A165 centre (41.0613, -17.3733) radius 1.75
  line L79 (34.167, -17.1965) -> (33.8135, -16.8429)
  arc A166 (31.5378, -98.1221) -> (0, -78.3) centre (0, -113.3) ccw
  line L80 (11.5396, -39.8239) -> (39.8239, -11.5396)
  line L81 (34.167, -17.1965) -> (33.8135, -16.8429)
  circle A167 centre (41.0613, -17.3733) radius 1.75
  arc A168 (35.2806, 96.2368) -> (0, 102.5) centre (0, 0) ccw
  arc A169 (35.2806, 96.2368) -> (0, 102.5) centre (0, 0) ccw
  line L82 (34.167, -17.1965) -> (33.8135, -16.8429)
  circle A170 centre (41.0613, -17.3733) radius 1.75
  line L83 (65.6333, -59.9764) -> (59.9764, -65.6333)
  line L84 (72.7044, -74.1186) -> (67.7546, -69.1688)
  line L85 (-17.1965, 34.167) -> (-16.8429, 33.8135)
  line L86 (65.6333, -59.9764) -> (59.9764, -65.6333)
  line L87 (-49.7234, 68.8153) -> (-68.8153, 49.7234)
  line L88 (72.7044, -74.1186) -> (70.2295, -71.6437)
  line L89 (-33.8135, 84.7252) -> (-37.0951, 88.0068)
  line L90 (49.0163, -92.8569) -> (42.807, -86.6476)
  line L91 (72.7044, -74.1186) -> (67.7546, -69.1688)
  line L92 (-30.5907, -80.8769) -> (-77.6541, -33.8135)
  line L93 (-51.8447, -34.8741) -> (-34.8741, -51.8447)
  line L94 (74.1186, -72.7044) -> (72.7044, -74.1186)
  line L95 (69.1688, -67.7546) -> (74.1186, -72.7044)
  line L96 (17.1965, 34.167) -> (16.8429, 33.8135)
  line L97 (72.7044, -74.1186) -> (67.7546, -69.1688)
  line L98 (72.7044, -74.1186) -> (67.7546, -69.1688)
  line L99 (-77.6541, 33.8135) -> (-33.8135, 77.6541)
  line L100 (-49.7234, 68.8153) -> (-68.8153, 49.7234)
  line L101 (74.1186, -72.7044) -> (72.7044, -74.1186)
  arc A171 (40.8846, -77.6541) -> (40.8846, -84.7252) centre (44.4201, -81.1896) ccw
  line L102 (-77.6541, 33.8135) -> (-33.8135, 77.6541)
  line L103 (74.1186, -72.7044) -> (72.7044, -74.1186)
  line L104 (-51.8447, -34.8741) -> (-34.8741, -51.8447)
  line L105 (-70.9366, 70.9366) -> (-49.0163, 92.8569)
  line L106 (-37.7026, 56.7945) -> (-49.7234, 68.8153)
  line L107 (56.4409, -62.0978) -> (40.8846, -77.6541)
  line L108 (59.9764, -65.6333) -> (56.4409, -62.0978)
  arc A172 (40.8846, -77.6541) -> (40.8846, -84.7252) centre (44.4201, -81.1896) ccw
  line L109 (-38.7632, -55.7338) -> (-55.7338, -38.7632)
  circle A173 centre (-17.3733, 41.0613) radius 1.75
  circle A174 centre (17.3733, 41.0613) radius 1.75
  line L110 (72.7044, -74.1186) -> (70.2295, -71.6437)
  line L111 (49.7234, -68.8153) -> (37.7026, -56.7945)
  line L112 (56.4409, -62.0978) -> (62.0978, -56.4409)
  line L113 (69.1688, -67.7546) -> (74.1186, -72.7044)
  line L114 (49.7234, -68.8153) -> (37.7026, -56.7945)
  line L115 (-62.0978, 56.4409) -> (-77.6541, 40.8846)
  line L116 (49.7234, -68.8153) -> (37.7026, -56.7945)
  line L117 (-62.0978, 56.4409) -> (-77.6541, 40.8846)
  line L118 (-37.7026, 56.7945) -> (-49.7234, 68.8153)
  line L119 (-16.8429, 33.8135) -> (-33.8135, 16.8429)
  line L120 (-56.4409, -62.0978) -> (-40.8846, -77.6541)
  line L121 (17.1965, 34.167) -> (16.8429, 33.8135)
  line L122 (-62.0978, 56.4409) -> (-77.6541, 40.8846)
  line L123 (56.4409, -62.0978) -> (62.0978, -56.4409)
  circle A175 centre (-17.3733, 41.0613) radius 1.75
  line L124 (37.5772, -88.4889) -> (40.3326, -91.2443)
  line L125 (49.7234, -68.8153) -> (37.7026, -56.7945)
  line L126 (59.9764, -65.6333) -> (56.4409, -62.0978)
  line L127 (74.1186, -72.7044) -> (72.7044, -74.1186)
  line L128 (49.0163, -92.8569) -> (70.9366, -70.9366)
  line L129 (-49.7234, -68.8153) -> (-37.7026, -56.7945)
  line L130 (-56.7945, 37.7026) -> (-37.7026, 56.7945)
  line L131 (-41.5917, -85.4323) -> (-49.0163, -92.8569)
  line L132 (-37.7026, -56.7945) -> (-56.7945, -37.7026)
  line L133 (-17.1965, 34.167) -> (-16.8429, 33.8135)
  line L134 (59.9764, -65.6333) -> (56.4409, -62.0978)
  circle A176 centre (17.3733, 41.0613) radius 1.75
  line L135 (56.4409, -62.0978) -> (40.8846, -77.6541)
  line L136 (69.1688, -67.7546) -> (74.1186, -72.7044)
  line L137 (59.9764, -65.6333) -> (56.4409, -62.0978)
  line L138 (-37.7026, -56.7945) -> (-56.7945, -37.7026)
  line L139 (41.5917, -85.4323) -> (49.0163, -92.8569)
  arc A177 (37.7434, -95.2979) -> (39.6929, -94.5025) centre (0, 0) ccw
  line L140 (-57.5016, -29.2173) -> (-29.2173, -57.5016)
  line L141 (-29.2173, 57.5016) -> (-57.5016, 29.2173)
  line L142 (68.8153, -49.7234) -> (49.7234, -68.8153)
  arc A178 (-97.869, 44.4738) -> (-97.869, -44.4738) centre (0, 0) ccw
  arc A179 (97.869, -44.4738) -> (97.869, 44.4738) centre (0, 0) ccw
  line L143 (-57.5016, 29.2173) -> (-39.8239, 11.5396)
  line L144 (37.7026, -56.7945) -> (56.7945, -37.7026)
  line L145 (39.8239, -11.5396) -> (57.5016, -29.2173)
  line L146 (68.8153, -49.7234) -> (49.7234, -68.8153)
  line L147 (51.8447, 34.8741) -> (55.7338, 38.7632)
  line L148 (37.7026, -56.7945) -> (56.7945, -37.7026)
  line L149 (-37.7026, -56.7945) -> (-56.7945, -37.7026)
  line L150 (-49.7234, 68.8153) -> (-68.8153, 49.7234)
  line L151 (56.4409, -62.0978) -> (62.0978, -56.4409)
  line L152 (30.5907, -80.8769) -> (77.6541, -33.8135)
  line L153 (65.6333, -59.9764) -> (59.9764, -65.6333)
  arc A180 (-96.2368, 35.2806) -> (-96.2368, -35.2806) centre (0, 0) ccw
  line L154 (-39.8239, 11.5396) -> (-11.5396, 39.8239)
  circle A181 centre (51.6679, -27.9799) radius 1.75
  line L155 (-37.7026, -56.7945) -> (-56.7945, -37.7026)
  line L156 (57.5016, -29.2173) -> (29.2173, -57.5016)
  line L157 (57.5016, -29.2173) -> (29.2173, -57.5016)
  line L158 (57.5016, -29.2173) -> (29.2173, -57.5016)
  line L159 (-70.9366, 70.9366) -> (-49.0163, 92.8569)
  line L160 (65.6333, -59.9764) -> (59.9764, -65.6333)
  circle A182 centre (-41.0613, -17.3733) radius 1.75
  line L161 (-56.7945, 37.7026) -> (-37.7026, 56.7945)
  line L162 (-39.8239, -11.5396) -> (-57.5016, -29.2173)
  line L163 (56.4409, -62.0978) -> (62.0978, -56.4409)
  circle A183 centre (51.6679, -27.9799) radius 1.75
  line L164 (49.0163, -92.8569) -> (70.9366, -70.9366)
  line L165 (-41.5917, -85.4323) -> (-49.0163, -92.8569)
  line L166 (70.9366, -70.9366) -> (92.8569, -49.0163)
  circle A184 centre (-41.0613, 17.3733) radius 1.75
  arc A185 (97.869, -44.4738) -> (97.869, 44.4738) centre (0, 0) ccw
  line L167 (-56.7945, 37.7026) -> (-37.7026, 56.7945)
  circle A186 centre (51.6679, -27.9799) radius 1.75
  line L168 (30.5907, -80.8769) -> (77.6541, -33.8135)
  line L169 (56.7945, -37.7026) -> (68.8153, -49.7234)
  line L170 (68.8153, -49.7234) -> (49.7234, -68.8153)
  line L171 (68.8153, -49.7234) -> (49.7234, -68.8153)
  line L172 (56.7945, -37.7026) -> (68.8153, -49.7234)
  line L173 (-49.7234, -68.8153) -> (-37.7026, -56.7945)
  line L174 (56.7945, -37.7026) -> (68.8153, -49.7234)
  line L175 (-56.7945, 37.7026) -> (-37.7026, 56.7945)
  line L176 (57.5016, -29.2173) -> (29.2173, -57.5016)
  line L177 (37.7026, -56.7945) -> (56.7945, -37.7026)
  line L178 (-39.8239, -11.5396) -> (-57.5016, -29.2173)
  line L179 (-29.2173, 57.5016) -> (-57.5016, 29.2173)
  line L180 (-49.7234, 68.8153) -> (-68.8153, 49.7234)
  line L181 (39.8239, -11.5396) -> (57.5016, -29.2173)
  arc A187 (-97.869, 44.4738) -> (-97.869, -44.4738) centre (0, 0) ccw
  arc A188 (-99.7259, 40.1371) -> (-99.7259, -40.1371) centre (0, 0) ccw
  line L182 (37.7026, -56.7945) -> (56.7945, -37.7026)
  line L183 (70.9366, -70.9366) -> (92.8569, -49.0163)
  line L184 (56.7945, -37.7026) -> (68.8153, -49.7234)
  circle A189 centre (-41.0613, 17.3733) radius 1.75
  arc A190 (24.049, -81.3368) -> (30.5907, -80.8769) centre (27.0551, -77.3414) ccw
  line L185 (33.8135, -16.8429) -> (16.8429, -33.8135)
  line L186 (51.8447, -34.8741) -> (34.8741, -51.8447)
  arc A191 (40.1371, 99.7259) -> (-40.1371, 99.7259) centre (0, 0) ccw
  line L187 (29.2173, -57.5016) -> (11.5396, -39.8239)
  line L188 (86.1394, 35.2277) -> (84.7252, 33.8135)
  circle A192 centre (27.9799, 51.6679) radius 1.75
  line L189 (17.1965, -34.167) -> (34.167, -17.1965)
  line L190 (51.8447, -34.8741) -> (34.8741, -51.8447)
  line L191 (11.5396, -39.8239) -> (39.8239, -11.5396)
  arc A193 (31.5378, -98.1221) -> (0, -78.3) centre (0, -113.3) ccw
  line L192 (33.8135, -16.8429) -> (16.8429, -33.8135)
  line L193 (16.8429, 33.8135) -> (33.8135, 16.8429)
  circle A194 centre (27.9799, 51.6679) radius 1.75
  line L194 (51.8447, 34.8741) -> (55.7338, 38.7632)
  line L195 (34.8741, -51.8447) -> (38.7632, -55.7338)
  line L196 (29.2173, 57.5016) -> (57.5016, 29.2173)
  arc A195 (-96.2368, 35.2806) -> (-96.2368, -35.2806) centre (0, 0) ccw
  line L197 (11.5396, -39.8239) -> (39.8239, -11.5396)
  circle A196 centre (-41.0613, 17.3733) radius 1.75
  line L198 (29.2173, 57.5016) -> (57.5016, 29.2173)
  line L199 (-57.5016, 29.2173) -> (-39.8239, 11.5396)
  circle A197 centre (-41.0613, 17.3733) radius 1.75
  circle A198 centre (27.9799, -51.6679) radius 1.75
  line L200 (34.8741, -51.8447) -> (38.7632, -55.7338)
  line L201 (33.8135, -16.8429) -> (16.8429, -33.8135)
  line L202 (39.8239, -11.5396) -> (57.5016, -29.2173)
  line L203 (77.6541, 33.8135) -> (33.8135, 77.6541)
  line L204 (34.8741, -51.8447) -> (38.7632, -55.7338)
  arc A199 (96.2368, -35.2806) -> (96.2368, 35.2806) centre (0, 0) ccw
  circle A200 centre (27.9799, -51.6679) radius 1.75
  line L205 (17.1965, -34.167) -> (34.167, -17.1965)
  line L206 (86.1394, 35.2277) -> (84.7252, 33.8135)
  line L207 (29.2173, -57.5016) -> (11.5396, -39.8239)
  line L208 (38.7632, -55.7338) -> (55.7338, -38.7632)
  line L209 (38.7632, -55.7338) -> (55.7338, -38.7632)
  line L210 (51.8447, -34.8741) -> (34.8741, -51.8447)
  line L211 (29.2173, -57.5016) -> (11.5396, -39.8239)
  line L212 (38.7632, -55.7338) -> (55.7338, -38.7632)
  line L213 (33.8135, -16.8429) -> (16.8429, -33.8135)
  line L214 (11.5396, 39.8239) -> (29.2173, 57.5016)
  line L215 (51.8447, -34.8741) -> (34.8741, -51.8447)
  arc A201 (96.2368, -35.2806) -> (96.2368, 35.2806) centre (0, 0) ccw
  line L216 (39.8239, 11.5396) -> (11.5396, 39.8239)
  line L217 (77.6541, 33.8135) -> (33.8135, 77.6541)
  arc A202 (-97.869, 44.4738) -> (-97.869, -44.4738) centre (0, 0) ccw
  arc A203 (44.4738, 97.869) -> (0, 107.5) centre (0, 0) ccw
  line L218 (11.5396, -39.8239) -> (39.8239, -11.5396)
  circle A204 centre (51.6679, -27.9799) radius 1.75
  line L219 (55.7338, -38.7632) -> (51.8447, -34.8741)
  line L220 (-57.5016, 29.2173) -> (-39.8239, 11.5396)
  arc A205 (99.7259, -40.1371) -> (99.7259, 40.1371) centre (0, 0) ccw
  line L221 (-57.5016, 29.2173) -> (-39.8239, 11.5396)
  line L222 (39.8239, -11.5396) -> (57.5016, -29.2173)
  arc A206 (-97.869, 44.4738) -> (-97.869, -44.4738) centre (0, 0) ccw
  arc A207 (-96.2368, 35.2806) -> (-96.2368, -35.2806) centre (0, 0) ccw
  arc A208 (-96.2368, 35.2806) -> (-96.2368, -35.2806) centre (0, 0) ccw
  line L223 (-39.8239, 11.5396) -> (-11.5396, 39.8239)
  line L224 (17.1965, -34.167) -> (34.167, -17.1965)
  line L225 (55.7338, -38.7632) -> (51.8447, -34.8741)
  line L226 (34.8741, -51.8447) -> (38.7632, -55.7338)
  arc A209 (-40.1371, -99.7259) -> (40.1371, -99.7259) centre (0, 0) ccw
  line L227 (11.5396, 39.8239) -> (29.2173, 57.5016)
  line L228 (55.7338, -38.7632) -> (51.8447, -34.8741)
  line L229 (39.8239, 11.5396) -> (11.5396, 39.8239)
  line L230 (38.7632, -55.7338) -> (55.7338, -38.7632)
  line L231 (55.7338, -38.7632) -> (51.8447, -34.8741)
  line L232 (17.1965, -34.167) -> (34.167, -17.1965)
  arc A210 (44.4738, 97.869) -> (0, 107.5) centre (0, 0) ccw
  circle A211 centre (27.9799, -51.6679) radius 1.75
  line L233 (16.8429, 33.8135) -> (33.8135, 16.8429)
  line L234 (65.6333, 59.9764) -> (62.0978, 56.4409)
  line L235 (67.7546, 69.1688) -> (72.7044, 74.1186)
  circle A212 centre (64.2191, 64.2191) radius 1
  arc A213 (47.1639, 91.0045) -> (46.9055, 91.138) centre (0, 0) ccw
  arc A214 (47.1639, 91.0045) -> (46.9055, 91.138) centre (0, 0) ccw
  line L236 (72.7044, 74.1186) -> (74.1186, 72.7044)
  line L237 (49.7234, 68.8153) -> (40.8846, 77.6541)
  line L238 (37.7026, 56.7945) -> (49.7234, 68.8153)
  arc A215 (42.807, 86.6476) -> (40.1371, 99.7259) centre (37.1501, 92.3045) ccw
  line L239 (56.7945, 37.7026) -> (37.7026, 56.7945)
  line L240 (56.7945, 37.7026) -> (37.7026, 56.7945)
  line L241 (37.7026, 56.7945) -> (49.7234, 68.8153)
  line L242 (49.0163, 92.8569) -> (40.8846, 84.7252)
  line L243 (49.0163, 92.8569) -> (42.807, 86.6476)
  line L244 (49.0163, 92.8569) -> (40.8846, 84.7252)
  line L245 (33.8135, 16.8429) -> (34.167, 17.1965)
  line L246 (83.0899, 32.1782) -> (81.1896, 30.278)
  line L247 (80.8769, 30.5907) -> (81.1896, 30.278)
  circle A216 centre (51.6679, 27.9799) radius 1.75
  line L248 (57.5016, 29.2173) -> (39.8239, 11.5396)
  circle A217 centre (41.0613, 17.3733) radius 1.75
  line L249 (57.5016, 29.2173) -> (39.8239, 11.5396)
  circle A218 centre (41.0613, 17.3733) radius 1.75
  line L250 (83.0899, 32.1782) -> (81.1896, 30.278)
  arc A219 (77.6541, 33.8135) -> (84.7252, 33.8135) centre (81.1896, 37.349) ccw
  line L251 (88.4889, 37.5772) -> (86.1394, 35.2277)
  line L252 (85.4323, 41.5917) -> (92.8569, 49.0163)
  line L253 (92.8569, 49.0163) -> (86.6476, 42.807)
  line L254 (85.4323, 41.5917) -> (84.7252, 40.8846)
  arc A220 (96.2368, 35.2806) -> (88.0068, 37.0951) centre (91.5424, 33.5596) ccw
  line L255 (85.4323, 41.5917) -> (92.8569, 49.0163)
  line L256 (85.4323, 41.5917) -> (84.7252, 40.8846)
  arc A221 (97.869, 44.4738) -> (89.7814, 45.9408) centre (93.3169, 42.4052) ccw
  arc A222 (97.869, 44.4738) -> (89.7814, 45.9408) centre (93.3169, 42.4052) ccw
  line L257 (68.8153, 49.7234) -> (56.7945, 37.7026)
  line L258 (62.0978, 56.4409) -> (77.6541, 40.8846)
  line L259 (62.0978, 56.4409) -> (77.6541, 40.8846)
  line L260 (68.8153, 49.7234) -> (56.7945, 37.7026)
  line L261 (56.4409, 62.0978) -> (59.9764, 65.6333)
  line L262 (67.0475, 69.8759) -> (69.8759, 67.0475)
  line L263 (92.8569, 49.0163) -> (70.9366, 70.9366)
  line L264 (49.7234, 68.8153) -> (68.8153, 49.7234)
  line L265 (59.9764, 65.6333) -> (65.6333, 59.9764)
  arc A223 (45.9408, 89.7814) -> (44.4738, 97.869) centre (42.4052, 93.3169) ccw
  line L266 (67.7546, 69.1688) -> (72.7044, 74.1186)
  line L267 (59.9764, 65.6333) -> (65.6333, 59.9764)
  line L268 (49.7234, 68.8153) -> (68.8153, 49.7234)
  line L269 (49.7234, 68.8153) -> (68.8153, 49.7234)